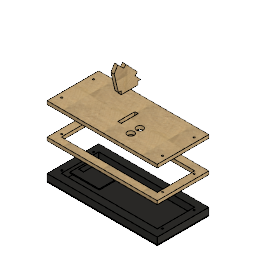
case (Autodesk Fusion 360 design; units mm, degrees)
Autodesk Fusion 360 part; units mm, degrees
sketch "Sketch1" plane through (0, 0, 0) normal (0, 0, 1) x (1, 0, 0) in component "top plate"
  line L0 (0, 0) -> (196, 0)
  line L1 (196, 0) -> (196, 92)
  line L2 (196, 92) -> (0, 92)
  line L3 (0, 92) -> (0, 0)
  dimension "d1" = 196
  dimension "d2" = 92
  constraint horizontal L0
  constraint vertical L1
  constraint horizontal L2
  constraint vertical L3
  constraint coincident L0.start L3.end
  measures "d1" distance of L0.start L0.end
  measures "d2" distance of L0.start L2.end
extrude "Extrude1" add sketch "Sketch1" along normal blind 1.6 makes body 1 in component "top plate"
sketch "Sketch1 (2)" plane through (0, 0, 1.6) normal (0, 0, 1) x (-1, 0, 0) in component "mid"
  line L0 (0, -92) -> (0, 0)
  line L1 (0, 0) -> (-196, 0)
  line L2 (-196, 0) -> (-196, -92)
  line L3 (-196, -92) -> (0, -92)
  line L4 (0, 0) -> (-196, 0)
  line L5 (-196, 0) -> (-196, -92)
  line L6 (-196, -92) -> (0, -92)
  line L7 (0, -92) -> (0, 0)
  line L8 (-12.8, -12.8) -> (-183.2, -12.8)
  line L9 (-183.2, -12.8) -> (-183.2, -79.2)
  line L10 (-183.2, -79.2) -> (-12.8, -79.2)
  line L11 (-12.8, -79.2) -> (-12.8, -12.8)
  dimension "d26" = -12.8
  constraint horizontal L4
  constraint vertical L5
  constraint horizontal L6
  constraint vertical L7
  constraint coincident L2.end L3.start
  constraint coincident L0.end L1.start
extrude "Extrude1'" add sketch "Sketch1 (2)" along normal blind 12 separate body makes body 2 in component "mid"
sketch "Sketch2" plane through (0, 0, 13.6) normal (0, 0, 1) x (-1, 0, 0) in component "mid"
  line L0 (-12.8, -12.8) -> (-12.8, -79.2)
  line L1 (-12.8, -79.2) -> (-183.2, -79.2)
  line L2 (-183.2, -79.2) -> (-183.2, -12.8)
  line L3 (-183.2, -12.8) -> (-12.8, -12.8)
  line L4 (0, -92) -> (0, 0)
  line L5 (0, 0) -> (-196, 0)
  line L6 (-196, 0) -> (-196, -92)
  line L7 (-196, -92) -> (0, -92)
  circle A0 centre (-8.6, -74.2) radius 1.5
  circle A1 centre (-8.6, -17.8) radius 1.5
  circle A2 centre (-187.4, -74.2) radius 1.5
  circle A3 centre (-187.4, -17.8) radius 1.5
  dimension "d29" = 3
  dimension "d30" = 17.8
  dimension "d31" = 8.6
  dimension "d32" = 17.8
  dimension "d33" = 8.6
  constraint vertical A0.centre A1.centre
  constraint horizontal A0.centre A2.centre
  constraint vertical A2.centre A3.centre
  constraint horizontal A1.centre A3.centre
  constraint equal A0 A2
  constraint equal A2 A3
  constraint equal A1 A3
  measures "d29" diameter of A0
  measures "d30" distance of L7 A0.centre
  measures "d31" distance of L4 A0.centre
  measures "d32" distance of L5 A1.centre
  measures "d33" distance of L6 A2.centre
extrude "Extrude2" cut sketch "Sketch2" against normal up to surface (12 mm away) contours A0 | A1 | A2 | A3 bodies 2 in component "mid"
sketch "Sketch1 (3)" plane through (0, 0, 1.6) normal (0, 0, 1) x (-1, 0, 0) in component "components"
  line L0 (0, -92) -> (0, 0)
  line L1 (0, 0) -> (-196, 0)
  line L2 (-196, 0) -> (-196, -92)
  line L3 (-196, -92) -> (0, -92)
  line L4 (-22.5, -61.8) -> (-31, -61.8)
  line L5 (-31, -61.8) -> (-31, -34)
  line L6 (-31, -34) -> (-22.5, -34)
  line L7 (-22.5, -34) -> (-22.5, -61.8)
  dimension "d36" = 27.8
  dimension "d37" = 8.5
  dimension "d38" = 61.8
  dimension "d39" = 31
  constraint horizontal L4
  constraint vertical L5
  constraint horizontal L6
  constraint vertical L7
  measures "d36" distance of L4.start L6.end
  measures "d37" distance of L4.start L4.end
  measures "d38" distance of L1 L4
  measures "d39" distance of L0 L5
extrude "Extrude1''" add sketch "Sketch1 (3)" along normal blind 11.2 separate body contours L4 L5 L6 L7 makes body 3 in component "components"
sketch "Sketch1 (4)" plane through (0, 0, 12.8) normal (0, 0, 1) x (-1, 0, 0) in component "PCB"
  line L0 (-22.5, -34) -> (-31, -34)
  line L1 (-31, -34) -> (-31, -61.8)
  line L2 (-31, -61.8) -> (-22.5, -61.8)
  line L3 (-22.5, -61.8) -> (-22.5, -34)
  line L4 (-19.2027, -65.4556) -> (-71.2727, -65.4556)
  line L5 (-71.2727, -65.4556) -> (-71.2727, -21.6456)
  line L6 (-71.2727, -21.6456) -> (-19.2027, -21.6456)
  line L7 (-19.2027, -21.6456) -> (-19.2027, -65.4556)
  dimension "d42" = 52.07
  dimension "d43" = 43.81
  constraint horizontal L4
  constraint vertical L5
  constraint horizontal L6
  constraint vertical L7
  measures "d42" distance of L4.start L4.end
  measures "d43" distance of L4.start L6.end
extrude "Extrude2'" add sketch "Sketch1 (4)" along normal blind 1.6 separate body contours L0 L1 L2 L3 | L4 L5 L6 L7 makes body 4 in component "PCB"
extrude "Extrude1'''" add sketch "Sketch1 (4)" along normal blind 1.6 separate body makes body 5 in component "PCB"
sketch "Sketch1 (5)" plane through (0, 0, 13.6) normal (0, 0, 1) x (-1, 0, 0) in component "mid (1)"
  circle A0 centre (-187.4, -74.2) radius 1.5
  circle A1 centre (-8.6, -74.2) radius 1.5
  circle A2 centre (-187.4, -17.8) radius 1.5
  circle A3 centre (-8.6, -17.8) radius 1.5
  line L0 (-12.8, -12.8) -> (-12.8, -79.2)
  line L1 (-12.8, -79.2) -> (-183.2, -79.2)
  line L2 (-183.2, -79.2) -> (-183.2, -12.8)
  line L3 (-183.2, -12.8) -> (-12.8, -12.8)
  line L4 (0, -92) -> (0, 0)
  line L5 (0, 0) -> (-196, 0)
  line L6 (-196, 0) -> (-196, -92)
  line L7 (-196, -92) -> (0, -92)
  line L8 (0, -92) -> (-196, -92)
  line L9 (-196, -92) -> (-196, 0)
  line L10 (-196, 0) -> (0, 0)
  line L11 (0, 0) -> (0, -92)
  circle A4 centre (-8.6, -74.2) radius 1.5
  circle A5 centre (-8.6, -17.8) radius 1.5
  circle A6 centre (-187.4, -74.2) radius 1.5
  circle A7 centre (-187.4, -17.8) radius 1.5
  constraint horizontal L8
  constraint vertical L9
  constraint horizontal L10
  constraint vertical L11
  constraint coincident L5.end L6.start
  constraint coincident L4.start L7.end
  constraint equal A1 A4
  constraint concentric A1 A4
  constraint coincident A3.centre A5.centre
  constraint equal A3 A5
  constraint concentric A0 A6
  constraint equal A0 A6
  constraint concentric A2 A7
  constraint equal A2 A7
extrude "Extrude1''''" add sketch "Sketch1 (5)" along normal blind 6 separate body makes body 6 in component "mid (1)"
sketch "Sketch1 (6)" plane through (0, 0, 19.6) normal (0, 0, 1) x (-1, 0, 0) in component "cover"
  circle A0 centre (-187.4, -74.2) radius 1.5
  circle A1 centre (-187.4, -17.8) radius 1.5
  circle A2 centre (-8.6, -17.8) radius 1.5
  circle A3 centre (-8.6, -74.2) radius 1.5
  line L0 (0, 0) -> (-196, 0)
  line L1 (-196, 0) -> (-196, -92)
  line L2 (-196, -92) -> (0, -92)
  line L3 (0, -92) -> (0, 0)
  line L4 (-125, -111.1325) -> (-125, 40) construction
  circle A4 centre (-125, -40) radius 6
  circle A5 centre (-125, -24) radius 6
  dimension "d64" = 125
  dimension "d65" = 12
  dimension "d66" = 12
  dimension "d67" = 40
  dimension "d68" = 24
  dimension "d100" = 0
  dimension "d101" = 0
  dimension "d102" = 0
  dimension "d103" = 0
  dimension "d112" = 0
  dimension "d113" = 0
  dimension "d114" = 0
  dimension "d115" = 0
  dimension "d120" = 0
  dimension "d121" = 0
  dimension "d122" = 0
  dimension "d123" = 0
  dimension "d128" = 0
  dimension "d129" = 0
  dimension "d130" = 0
  dimension "d131" = 0
  constraint vertical L4
  constraint coincident L4 A4.centre
  constraint coincident L4 A5.centre
  measures "d64" distance of L3 L4
  measures "d65" diameter of A4
  measures "d66" diameter of A5
  measures "d67" distance of L0 A4.centre
  measures "d68" distance of L0 A5.centre
extrude "Extrude1'''''" add sketch "Sketch1 (6)" along normal blind 6 separate body makes body 7 in component "cover"
ref_plane "WorkPlane3" through (80, 46, 22.6) normal (-1, 0, 0) x (0, -1, 0) in component "leg"
sketch "Sketch6" plane through (0, 0, 0) normal (-1, 0, 0) x (0, -1, 0) in component "leg"
  line L0 (-92, 19.6) -> (0, 19.6)
  line L1 (0, 19.6) -> (0, 25.6)
  line L2 (0, 25.6) -> (-92, 25.6)
  line L3 (-92, 25.6) -> (-92, 19.6)
  line L4 (-66, 25.6) -> (-26, 25.6)
  line L5 (-61, 25.6) -> (-31, 25.6)
  line L6 (-31, 25.6) -> (-31, 19.6)
  line L7 (-31, 19.6) -> (-61, 19.6)
  line L8 (-61, 19.6) -> (-61, 25.6)
  line L9 (-26, 25.6) -> (-18.4045, 57.4776)
  line L10 (-18.4045, 57.4776) -> (-25.0186, 68.9335)
  line L11 (-25.0186, 68.9335) -> (-66, 25.6)
  line L12 (-78.4907, 12.3923) -> (-12.5279, 82.1412) construction
  line L13 (-55.816, 36.3685) -> (-35.2026, 58.165)
  line L14 (-35.2026, 58.165) -> (-39.5619, 62.2877)
  line L15 (-39.5619, 62.2877) -> (-60.1753, 40.4912)
  line L16 (-60.1753, 40.4912) -> (-55.816, 36.3685)
  dimension "d86" = 40
  dimension "d87" = 30
  dimension "d88" = 6
  dimension "d89" = 60
  dimension "d90" = 30
  dimension "d92" = 96
  dimension "d93" = 6
  constraint coincident L2 L4.start
  constraint coincident L2 L4.end
  constraint midpoint L2 L4
  constraint horizontal L5
  constraint vertical L6
  constraint horizontal L7
  constraint vertical L8
  constraint coincident L4 L5.start
  constraint coincident L2 L5.start
  constraint midpoint L4 L5
  constraint coincident L1.end L10
  constraint parallel L11 L12
  constraint midpoint L11 L12
  constraint coincident L9 L12.end
  constraint perpendicular L13 L14
  constraint parallel L13 L15
  constraint parallel L14 L16
  constraint coincident L11 L13.end
  constraint parallel L11 L13
  constraint midpoint L12 L13
  constraint equal L7 L15
  measures "d86" distance of L4.start L4.end
  measures "d87" distance of L5.start L5.end
  measures "d88" distance of L5.start L7.end
  measures "d89" angle of L4 L10
  measures "d90" angle of L9 L11
  measures "d92" distance of L12.start L12.end
  measures "d93" distance of L13.end L14.end
extrude "Extrude1''''''" add sketch "Sketch6" against normal blind 6 separate body contours L0 L2 L4 L5 L6 L7 L8 | L2 L4 L5 L9 L10 L11 L13 | L11 L13 L14 L15 L16 makes body 8 in component "leg"
combine "Combine1" operation cut target body 7 tool bodies 8 body 8 seen with x (1, 0, 0) y (0, 1, 0) z (0, 0, 1) at (95, 0, 0) keep tools in component "cover"
sketch "mid_toDXF" plane through (0, 0, 64.3954) normal (0, 0, 1) x (-1, 0, 0)
  circle A0 centre (-164.0067, -113.7731) radius 1.5
  circle A1 centre (-164.0067, -57.3731) radius 1.5
  circle A2 centre (14.7933, -57.3731) radius 1.5
  circle A3 centre (14.7933, -113.7731) radius 1.5
  line L0 (-159.8067, -118.7731) -> (-159.8067, -52.3731)
  line L1 (-159.8067, -52.3731) -> (10.5933, -52.3731)
  line L2 (10.5933, -52.3731) -> (10.5933, -118.7731)
  line L3 (10.5933, -118.7731) -> (-159.8067, -118.7731)
  line L4 (23.3933, -39.5731) -> (-172.6067, -39.5731)
  line L5 (-172.6067, -39.5731) -> (-172.6067, -131.5731)
  line L6 (-172.6067, -131.5731) -> (23.3933, -131.5731)
  line L7 (23.3933, -131.5731) -> (23.3933, -39.5731)
sketch "cover_toDXF" plane through (0, 0, 120.3954) normal (0, 0, 1) x (-1, 0, 0)
  line L0 (-71.6067, -100.5731) -> (-77.6067, -100.5731)
  line L1 (-77.6067, -100.5731) -> (-77.6067, -70.5731)
  line L2 (-77.6067, -70.5731) -> (-71.6067, -70.5731)
  line L3 (-71.6067, -70.5731) -> (-71.6067, -100.5731)
  circle A0 centre (-101.6067, -79.5731) radius 6
  circle A1 centre (-101.6067, -63.5731) radius 6
  circle A2 centre (-164.0067, -57.3731) radius 1.5
  circle A3 centre (14.7933, -57.3731) radius 1.5
  circle A4 centre (14.7933, -113.7731) radius 1.5
  circle A5 centre (-164.0067, -113.7731) radius 1.5
  line L4 (23.3933, -131.5731) -> (23.3933, -39.5731)
  line L5 (23.3933, -39.5731) -> (-172.6067, -39.5731)
  line L6 (-172.6067, -39.5731) -> (-172.6067, -131.5731)
  line L7 (-172.6067, -131.5731) -> (23.3933, -131.5731)
sketch "leg_toDXF" plane through (71.6067, 0, 0) normal (-1, 0, 0) x (0, -1, 0)
  line L0 (-70.5731, 166.3954) -> (-65.5731, 166.3954)
  line L1 (-65.5731, 166.3954) -> (-57.9776, 198.2729)
  line L2 (-57.9776, 198.2729) -> (-64.5918, 209.7289)
  line L3 (-64.5918, 209.7289) -> (-74.7757, 198.9604)
  line L4 (-74.7757, 198.9604) -> (-79.1351, 203.0831)
  line L5 (-79.1351, 203.0831) -> (-99.7484, 181.2866)
  line L6 (-99.7484, 181.2866) -> (-95.3891, 177.1639)
  line L7 (-95.3891, 177.1639) -> (-105.5731, 166.3954)
  line L8 (-105.5731, 166.3954) -> (-100.5731, 166.3954)
  line L9 (-100.5731, 166.3954) -> (-100.5731, 160.3954)
  line L10 (-100.5731, 160.3954) -> (-70.5731, 160.3954)
  line L11 (-70.5731, 160.3954) -> (-70.5731, 166.3954)
extrude "Extrude2''" [suppressed] in component "mid (1)"
extrude "Extrude4" [suppressed] in component "mid (1)"
extrude "Extrude3" [suppressed] in component "mid (1)"
sketch "Sketch2 (2)" plane through (0, 0, 1.6) normal (0, 0, 1) x (-1, 0, 0) in component "top plate"
  line L0 (0, -92) -> (0, 0)
  line L1 (0, 0) -> (-196, 0)
  line L2 (-196, 0) -> (-196, -92)
  line L3 (-196, -92) -> (0, -92)
  line L4 (-2.5, -0.5) -> (-0.5, -0.5)
  line L5 (-0.5, -0.5) -> (-0.5, -2.5)
  line L6 (-0.5, -2.5) -> (-2.5, -2.5)
  line L7 (-2.5, -2.5) -> (-2.5, -0.5)
  line L8 (-2.5, -0.5) -> (-0.5, -2.5) construction
  line L9 (-0.5, -0.5) -> (-2.5, -2.5) construction
  point P0 (-1.5, -1.5)
  dimension "d5" = 2
  dimension "d6" = 2
  dimension "d7" = 1.5
  dimension "d8" = 1.5
  constraint perpendicular L4 L5
  constraint parallel L4 L6
  constraint parallel L5 L7
  constraint horizontal L4
  constraint coincident L8 P0
  constraint coincident L9 P0
  measures "d5" distance of L5.end L6.end
  measures "d6" distance of L4.end L5.end
  measures "d7" distance of L0 P0
  measures "d8" distance of L1 P0
extrude "Extrude2'''" [suppressed] in component "top plate"
component "display" placed x (1, 0, 0) y (0, 1, 0) z (0, 0, 1) at (0, 0, 0)
component "case" placed x (1, 0, 0) y (0, 1, 0) z (0, 0, 1) at (0, 0, 0)
component "top plate" placed x (1, 0, 0) y (0, 1, 0) z (0, 0, 1) at (-23.3933, 39.5731, -5.2046) in component "display"
component "mid" placed x (1, 0, 0) y (0, 1, 0) z (0, 0, 1) at (-23.3933, 39.5731, -5.2046) in component "display"
component "components" placed x (1, 0, 0) y (0, 1, 0) z (0, 0, 1) at (-23.3933, 39.5731, -5.2046) in component "display"
component "PCB" placed x (1, 0, 0) y (0, 1, 0) z (0, 0, 1) at (-23.3933, 39.5731, -5.2046) in component "display"
component "mid (1)" placed x (1, 0, 0) y (0, 1, 0) z (0, 0, 1) at (-23.3933, 39.5731, 44.7954) in component "case"
component "cover" placed x (1, 0, 0) y (0, 1, 0) z (0, 0, 1) at (-23.3933, 39.5731, 94.7954) in component "case"
component "leg" placed x (1, 0, 0) y (0, 1, 0) z (0, 0, 1) at (71.6067, 39.5731, 140.7954) in component "case"
component "leg" placed x (-1, 0, 0) y (0, 0.687113, -0.726551) z (0, -0.726551, -0.687113) at (77.6067, 88.6448, 185.9378) in component "case"
equation "pixel_pitch = 3 mm"
equation "matrix_width = 64"
equation "matrix_height = 32"
equation "display_width = pixel_pitch * matrix_width"
equation "display_height = pixel_pitch * matrix_height"
equation "thickness = 6 mm"
equation "d49 = thickness"
equation "d51 = thickness"
equation "socket_hole_diameter = 12 mm"
equation "cable_hole_diameter = 12 mm"
equation "d65 = socket_hole_diameter"
equation "d66 = cable_hole_diameter"
equation "d69 = thickness"
equation "d88 = thickness"
equation "d92 = display_height"
equation "d93 = thickness"
equation "d94 = -thickness"
